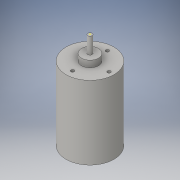
# Autodesk Inventor part: motor MABCHI 3W Noah
Saved by Autodesk Inventor 2016 (Build 200138000, 138)
## iProperties
Created: 2016-11-30
Part Number: motor MABCHI 3W Noah
Material: Generic
Document SubType Name: Modeling
Designer: Student
Density: 1 g/cm^3
Appearance: Default
Author: Student
Autodesk Inventor part; units mm, degrees
ref_plane "YZ Plane" through (0, 0, 0) normal (1, 0, 0) x (0, 1, 0)
ref_plane "XZ Plane" through (0, 0, 0) normal (0, 1, 0) x (-1, 0, 0)
ref_plane "XY Plane" through (0, 0, 0) normal (0, 0, 1) x (1, 0, 0)
sketch "Sketch1" plane through (0, 0, 0) normal (0, 1, 0) x (-1, 0, 0)
  circle A0 centre (0, 0) radius 18.6309
  dimension "d0" = 37.2618
  constraints: 1 centre point, 1 coincident
  measures "d0" diameter of A0
extrude "Extrusion1" add sketch "Sketch1" along normal blind 57.0738
sketch "Sketch2" plane through (0, 57.0738, 0) normal (0, 1, 0) x (1, 0, 0)
  circle A0 centre (0, 0) radius 6.604
  dimension "d3" = 13.208
  constraints: 1 centre point, 1 coincident
  measures "d3" diameter of A0
extrude "Extrusion2" add sketch "Sketch2" along normal blind 5.08
sketch "Sketch3" plane through (0, 57.0738, 0) normal (0, 1, 0) x (1, 0, 0)
  circle A0 centre (0, 13.5382) radius 1.27
  circle A1 centre (0, -13.5382) radius 1.2719
  circle A2 centre (14.8082, 0) radius 1.27
  point P0 (0, 0)
  dimension "d6" = 2.54
  dimension "d7" = 2.54
  dimension "d8" = 13.5382
  dimension "d9" = 13.5382
  dimension "d10" = 14.8082
  constraints: 3 centre point
  measures "d6" diameter of A0
  measures "d7" diameter of A2
  measures "d8" distance of point (0, 0) A0.centre
  measures "d9" distance of point (0, 0) A1.centre
  measures "d10" distance of point (0, 0) A2.centre
extrude "Extrusion3" cut sketch "Sketch3" against normal blind 76.2
sketch "Sketch4" plane through (0, 62.1538, 0) normal (0, 1, 0) x (1, 0, 0)
  circle A0 centre (0, 0) radius 1.7145
  dimension "d13" = 3.429
  constraints: 1 centre point, 1 coincident
  measures "d13" diameter of A0
extrude "Extrusion4" add sketch "Sketch4" along normal blind 12.7
sketch "Sketch5" plane through (0, 74.8538, 0) normal (0, 1, 0) x (1, 0, 0)
  point P0 (0, 0)
body "Solid1"
